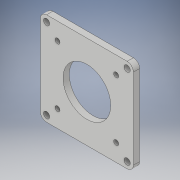
# Autodesk Inventor part: TurntableMotorBracket
Saved by Autodesk Inventor 2019.3 (Build 233278000, 278)
## iProperties
Created: 2019-07-07
Part Number: TurntableMotorBracket
Material: Generic
Document SubType Name: Modeling
Designer: mark
Density: 1 g/cm^3
Appearance: Default
Author: mark
Autodesk Inventor part; units mm, degrees
ref_plane "YZ Plane" through (0, 0, 0) normal (1, 0, 0) x (0, 1, 0)
ref_plane "XZ Plane" through (0, 0, 0) normal (0, 1, 0) x (-1, 0, 0)
ref_plane "XY Plane" through (0, 0, 0) normal (0, 0, 1) x (1, 0, 0)
sketch "Sketch1" plane through (0, 0, 0) normal (0, 0, 1) x (1, 0, 0)
  line L0 (-37.25, 37.25) -> (37.25, 37.25)
  line L1 (37.25, 37.25) -> (37.25, -37.25)
  line L2 (37.25, -37.25) -> (-37.25, -37.25)
  line L3 (-37.25, -37.25) -> (-37.25, 37.25)
  circle A0 centre (-23.5, 23.5) radius 2
  circle A1 centre (-23.5, -23.5) radius 2
  circle A2 centre (23.5, -23.5) radius 2
  circle A3 centre (23.5, 23.5) radius 2
  circle A4 centre (0, 0) radius 19.1
  circle A5 centre (-32.25, 32.25) radius 2.5
  circle A6 centre (32.25, 32.25) radius 2.5
  circle A7 centre (-32.25, -32.25) radius 2.5
  circle A8 centre (32.25, -32.25) radius 2.5
  dimension "d0" = 4
  dimension "d1" = 4
  dimension "d2" = 4
  dimension "d3" = 4
  dimension "d4" = 38.2
  dimension "d5" = 47
  dimension "d6" = 47
  dimension "d7" = 47
  dimension "d8" = 47
  dimension "d9" = 23.5
  dimension "d10" = 23.5
  dimension "d11" = 23.5
  dimension "d12" = 23.5
  dimension "d13" = 74.5
  dimension "d14" = 74.5
  dimension "d15" = 37.25
  dimension "d16" = 37.25
  dimension "d17" = 5
  dimension "d18" = 5
  dimension "d19" = 5
  dimension "d20" = 5
  dimension "d21" = 64.5
  dimension "d22" = 64.5
  dimension "d23" = 64.5
  dimension "d24" = 64.5
  dimension "d25" = 5
  dimension "d26" = 5
  dimension "d27" = 5
  dimension "d28" = 5
  constraints: 9 centre point, 8 end point, 2 horizontal, 2 vertical, 1 coincident
  measures "d0" diameter of A0
  measures "d1" diameter of A1
  measures "d2" diameter of A2
  measures "d3" diameter of A3
  measures "d4" diameter of A4
  measures "d5" distance of A3.centre A0.centre
  measures "d6" distance of A1.centre A0.centre
  measures "d7" distance of A1.centre A2.centre
  measures "d8" distance of A2.centre A3.centre
  measures "d9" horizontal distance of A3.centre point (0, 0)
  measures "d10" horizontal distance of point (0, 0) A3.centre
  measures "d11" horizontal distance of point (0, 0) A1.centre
  measures "d12" horizontal distance of A1.centre point (0, 0)
  measures "d13" distance between parallel lines of L1 L3
  measures "d14" distance between parallel lines of L2 L0
  measures "d15" distance from line of L2 point (0, 0)
  measures "d16" distance from line of L3 point (0, 0)
  measures "d17" diameter of A5
  measures "d18" diameter of A6
  measures "d19" diameter of A7
  measures "d20" diameter of A8
  measures "d21" distance of A6.centre A5.centre
  measures "d22" distance of A7.centre A5.centre
  measures "d23" distance of A8.centre A7.centre
  measures "d24" distance of A8.centre A6.centre
  measures "d25" distance from line of L1 A6.centre
  measures "d26" distance from line of L0 A6.centre
  measures "d27" distance from line of L2 A7.centre
  measures "d28" distance from line of L3 A7.centre
extrude "Extrusion1" add sketch "Sketch1" along normal blind 5
fillet "Fillet1" radius 5 4 edges at (37.25, 37.25, 2.5) (37.25, -37.25, 2.5) (-37.25, 37.25, 2.5) (-37.25, -37.25, 2.5)
body "Solid1"
